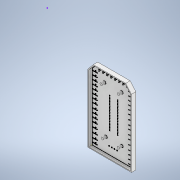
# Autodesk Inventor part: CaseV1
Saved by Autodesk Inventor 2021 (Build 250183000, 183)
## iProperties
Created: 2021-02-27
Part Number: CaseV1
Material: ABS Plastic
Document SubType Name: Modeling
Designer: Collin
Density: 1.06 g/cm^3
Appearance: Smooth - White
Mass: 45.9526 g
Surface Area: 316.416 cm^2
Volume: 43.3515 cm^3
Author: Collin
Autodesk Inventor part; units mm, degrees
ref_plane "YZ Plane" through (0, 0, 0) normal (1, 0, 0) x (0, 1, 0)
ref_plane "XZ Plane" through (0, 0, 0) normal (0, 1, 0) x (-1, 0, 0)
ref_plane "XY Plane" through (0, 0, 0) normal (0, 0, 1) x (1, 0, 0)
sketch "Sketch1" plane through (0, 0, 0) normal (0, 0, 1) x (1, 0, 0)
  line L0 (79.756, 127.254) -> (79.756, 0)
  line L1 (69.85, 138.938) -> (79.756, 127.254)
  line L2 (9.398, 138.938) -> (69.85, 138.938)
  line L3 (0, 127.762) -> (9.398, 138.938)
  line L4 (0, 0) -> (0, 127.762)
  line L5 (79.756, 0) -> (0, 0)
  circle A0 centre (28.448, 132.08) radius 0.51
  circle A1 centre (20.828, 132.08) radius 0.51
  circle A2 centre (22.988, 132.08) radius 0.55
  circle A3 centre (23.368, 115.57) radius 2.54
  circle A4 centre (13.208, 129.54) radius 0.51
  circle A5 centre (6.858, 101.6) radius 0.51
  circle A6 centre (9.398, 101.6) radius 0.51
  circle A7 centre (6.858, 103.76) radius 0.55
  circle A8 centre (9.398, 109.22) radius 0.51
  circle A9 centre (6.858, 109.22) radius 0.51
  circle A10 centre (6.858, 111.38) radius 0.55
  circle A11 centre (6.858, 124.46) radius 0.51
  circle A12 centre (9.398, 124.46) radius 0.51
  circle A13 centre (9.398, 116.84) radius 0.51
  circle A14 centre (6.858, 116.84) radius 0.51
  circle A15 centre (6.858, 119) radius 0.55
  circle A16 centre (6.858, 126.62) radius 0.55
  circle A17 centre (6.858, 96.14) radius 0.55
  circle A18 centre (6.858, 88.52) radius 0.55
  circle A19 centre (9.398, 93.98) radius 0.51
  circle A20 centre (6.858, 93.98) radius 0.51
  circle A21 centre (6.858, 39.37) radius 0.51
  circle A22 centre (6.858, 41.53) radius 0.55
  circle A23 centre (6.858, 49.15) radius 0.55
  circle A24 centre (6.858, 46.99) radius 0.51
  circle A25 centre (6.858, 54.61) radius 0.51
  circle A26 centre (6.858, 56.77) radius 0.55
  circle A27 centre (6.858, 80.9) radius 0.55
  circle A28 centre (6.858, 78.74) radius 0.51
  circle A29 centre (6.858, 73.28) radius 0.55
  circle A30 centre (6.858, 64.39) radius 0.55
  circle A31 centre (6.858, 71.12) radius 0.51
  circle A32 centre (6.858, 62.23) radius 0.51
  circle A33 centre (9.398, 71.12) radius 0.51
  circle A34 centre (9.398, 62.23) radius 0.51
  circle A35 centre (9.398, 39.37) radius 0.51
  circle A36 centre (9.398, 46.99) radius 0.51
  circle A37 centre (9.398, 54.61) radius 0.51
  circle A38 centre (9.398, 78.74) radius 0.51
  circle A39 centre (6.858, 86.36) radius 0.51
  circle A40 centre (9.398, 86.36) radius 0.51
  circle A41 centre (1.778, 78.74) radius 0.51
  circle A42 centre (1.778, 86.36) radius 0.51
  circle A43 centre (1.778, 109.22) radius 0.51
  circle A44 centre (1.778, 101.6) radius 0.51
  circle A45 centre (1.778, 93.98) radius 0.51
  circle A46 centre (4.318, 78.74) radius 0.51
  circle A47 centre (4.318, 86.36) radius 0.51
  circle A48 centre (4.318, 109.22) radius 0.51
  circle A49 centre (4.318, 101.6) radius 0.51
  circle A50 centre (4.318, 93.98) radius 0.51
  circle A51 centre (4.318, 39.37) radius 0.51
  circle A52 centre (1.778, 39.37) radius 0.51
  circle A53 centre (1.778, 54.61) radius 0.51
  circle A54 centre (4.318, 54.61) radius 0.51
  circle A55 centre (4.318, 46.99) radius 0.51
  circle A56 centre (1.778, 46.99) radius 0.51
  circle A57 centre (1.778, 71.12) radius 0.51
  circle A58 centre (4.318, 71.12) radius 0.51
  circle A59 centre (1.778, 62.23) radius 0.51
  circle A60 centre (4.318, 62.23) radius 0.51
  circle A61 centre (4.318, 124.46) radius 0.51
  circle A62 centre (4.318, 116.84) radius 0.51
  circle A63 centre (1.778, 116.84) radius 0.51
  circle A64 centre (1.778, 124.46) radius 0.51
  circle A65 centre (33.528, 40.64) radius 0.5
  circle A66 centre (36.068, 137.16) radius 0.51
  circle A67 centre (36.068, 134.62) radius 0.51
  circle A68 centre (36.068, 132.08) radius 0.51
  circle A69 centre (36.068, 129.54) radius 0.51
  circle A70 centre (33.528, 76.2) radius 0.5
  circle A71 centre (33.528, 78.74) radius 0.5
  circle A72 centre (33.528, 81.28) radius 0.5
  circle A73 centre (33.528, 88.9) radius 0.5
  circle A74 centre (33.528, 86.36) radius 0.5
  circle A75 centre (33.528, 83.82) radius 0.5
  circle A76 centre (33.528, 93.98) radius 0.5
  circle A77 centre (33.528, 91.44) radius 0.5
  circle A78 centre (33.528, 96.52) radius 0.5
  circle A79 centre (33.528, 99.06) radius 0.5
  circle A80 centre (33.528, 45.72) radius 0.5
  circle A81 centre (33.528, 48.26) radius 0.5
  circle A82 centre (33.528, 53.34) radius 0.5
  circle A83 centre (33.528, 50.8) radius 0.5
  circle A84 centre (33.528, 58.42) radius 0.5
  circle A85 centre (33.528, 55.88) radius 0.5
  circle A86 centre (33.528, 73.66) radius 0.5
  circle A87 centre (33.528, 71.12) radius 0.5
  circle A88 centre (33.528, 68.58) radius 0.5
  circle A89 centre (33.528, 63.5) radius 0.5
  circle A90 centre (33.528, 66.04) radius 0.5
  circle A91 centre (33.528, 60.96) radius 0.5
  circle A92 centre (30.608, 132.08) radius 0.55
  circle A93 centre (33.528, 43.18) radius 0.5
  circle A94 centre (13.208, 134.62) radius 0.51
  circle A95 centre (20.828, 134.62) radius 0.51
  circle A96 centre (15.368, 132.08) radius 0.55
  circle A97 centre (13.208, 132.08) radius 0.51
  circle A98 centre (20.828, 129.54) radius 0.51
  circle A99 centre (13.208, 137.16) radius 0.51
  circle A100 centre (20.828, 137.16) radius 0.51
  circle A101 centre (28.448, 137.16) radius 0.51
  circle A102 centre (28.448, 134.62) radius 0.51
  circle A103 centre (28.448, 129.54) radius 0.51
  circle A104 centre (77.978, 44.45) radius 0.51
  circle A105 centre (75.438, 46.61) radius 0.55
  circle A106 centre (75.438, 44.45) radius 0.51
  circle A107 centre (75.438, 54.23) radius 0.55
  circle A108 centre (75.438, 52.07) radius 0.51
  circle A109 centre (77.978, 52.07) radius 0.51
  circle A110 centre (77.978, 60.96) radius 0.51
  circle A111 centre (75.438, 60.96) radius 0.51
  circle A112 centre (75.438, 63.12) radius 0.55
  circle A113 centre (70.358, 52.07) radius 0.51
  circle A114 centre (70.358, 44.45) radius 0.51
  circle A115 centre (70.358, 60.96) radius 0.51
  circle A116 centre (72.898, 60.96) radius 0.51
  circle A117 centre (72.898, 44.45) radius 0.51
  circle A118 centre (72.898, 52.07) radius 0.51
  circle A119 centre (70.358, 68.326) radius 0.51
  circle A120 centre (72.898, 68.326) radius 0.51
  circle A121 centre (77.978, 68.326) radius 0.51
  circle A122 centre (75.438, 68.326) radius 0.51
  circle A123 centre (75.438, 79.376) radius 0.55
  circle A124 centre (75.438, 77.216) radius 0.51
  circle A125 centre (77.978, 77.216) radius 0.51
  circle A126 centre (75.438, 70.486) radius 0.55
  circle A127 centre (72.898, 77.216) radius 0.51
  circle A128 centre (70.358, 77.216) radius 0.51
  circle A129 centre (48.768, 78.74) radius 0.5
  circle A130 centre (48.768, 76.2) radius 0.5
  circle A131 centre (48.768, 73.66) radius 0.5
  circle A132 centre (48.768, 68.58) radius 0.5
  circle A133 centre (48.768, 71.12) radius 0.5
  circle A134 centre (48.768, 66.04) radius 0.5
  circle A135 centre (48.768, 50.8) radius 0.5
  circle A136 centre (48.768, 53.34) radius 0.5
  circle A137 centre (48.768, 58.42) radius 0.5
  circle A138 centre (48.768, 55.88) radius 0.5
  circle A139 centre (48.768, 63.5) radius 0.5
  circle A140 centre (48.768, 60.96) radius 0.5
  circle A141 centre (48.768, 48.26) radius 0.5
  circle A142 centre (48.768, 45.72) radius 0.5
  circle A143 centre (75.438, 103.506) radius 0.55
  circle A144 centre (75.438, 101.346) radius 0.51
  circle A145 centre (72.898, 101.346) radius 0.51
  circle A146 centre (75.438, 95.886) radius 0.55
  circle A147 centre (72.898, 86.106) radius 0.51
  circle A148 centre (75.438, 88.266) radius 0.55
  circle A149 centre (75.438, 86.106) radius 0.51
  circle A150 centre (75.438, 93.726) radius 0.51
  circle A151 centre (72.898, 93.726) radius 0.51
  circle A152 centre (70.358, 93.726) radius 0.51
  circle A153 centre (70.358, 101.346) radius 0.51
  circle A154 centre (70.358, 86.106) radius 0.51
  circle A155 centre (48.768, 86.36) radius 0.5
  circle A156 centre (48.768, 88.9) radius 0.5
  circle A157 centre (48.768, 91.44) radius 0.5
  circle A158 centre (48.768, 96.52) radius 0.5
  circle A159 centre (48.768, 93.98) radius 0.5
  circle A160 centre (48.768, 99.06) radius 0.5
  circle A161 centre (77.978, 93.726) radius 0.51
  circle A162 centre (77.978, 86.106) radius 0.51
  circle A163 centre (77.978, 101.346) radius 0.51
  circle A164 centre (48.768, 83.82) radius 0.5
  circle A165 centre (48.768, 81.28) radius 0.5
  circle A166 centre (66.548, 129.54) radius 0.51
  circle A167 centre (58.928, 129.54) radius 0.51
  circle A168 centre (51.308, 129.54) radius 0.51
  circle A169 centre (70.358, 123.952) radius 0.51
  circle A170 centre (72.898, 116.586) radius 0.51
  circle A171 centre (70.358, 116.586) radius 0.51
  circle A172 centre (72.898, 123.952) radius 0.51
  circle A173 centre (56.388, 115.57) radius 2.54
  circle A174 centre (77.978, 116.586) radius 0.51
  circle A175 centre (75.438, 116.586) radius 0.51
  circle A176 centre (75.438, 118.746) radius 0.55
  circle A177 centre (75.438, 126.112) radius 0.55
  circle A178 centre (75.438, 123.952) radius 0.51
  circle A179 centre (77.978, 123.952) radius 0.51
  circle A180 centre (75.438, 108.966) radius 0.51
  circle A181 centre (77.978, 108.966) radius 0.51
  circle A182 centre (72.898, 108.966) radius 0.51
  circle A183 centre (75.438, 111.126) radius 0.55
  circle A184 centre (70.358, 108.966) radius 0.51
  circle A185 centre (51.308, 137.16) radius 0.51
  circle A186 centre (51.308, 134.62) radius 0.51
  circle A187 centre (58.928, 137.16) radius 0.51
  circle A188 centre (58.928, 134.62) radius 0.51
  circle A189 centre (66.548, 134.62) radius 0.51
  circle A190 centre (66.548, 137.16) radius 0.51
  circle A191 centre (53.468, 132.08) radius 0.55
  circle A192 centre (61.088, 132.08) radius 0.55
  circle A193 centre (58.928, 132.08) radius 0.51
  circle A194 centre (51.308, 132.08) radius 0.51
  circle A195 centre (66.548, 132.08) radius 0.51
  circle A196 centre (68.708, 132.08) radius 0.55
  circle A197 centre (43.688, 129.54) radius 0.51
  circle A198 centre (43.688, 132.08) radius 0.51
  circle A199 centre (43.688, 134.62) radius 0.51
  circle A200 centre (45.848, 132.08) radius 0.55
  circle A201 centre (43.688, 137.16) radius 0.51
  circle A202 centre (48.768, 43.18) radius 0.5
  circle A203 centre (38.228, 132.08) radius 0.55
  circle A204 centre (48.768, 40.64) radius 0.5
  circle A205 centre (4.318, 12.7) radius 0.51
  circle A206 centre (6.858, 14.86) radius 0.55
  circle A207 centre (6.858, 12.7) radius 0.51
  circle A208 centre (9.398, 12.7) radius 0.51
  circle A209 centre (32.258, 14.732) radius 0.89
  circle A210 centre (37.338, 14.732) radius 0.89
  circle A211 centre (77.978, 19.05) radius 0.51
  circle A212 centre (75.438, 19.05) radius 0.51
  circle A213 centre (75.438, 13.59) radius 0.55
  circle A214 centre (70.358, 19.05) radius 0.51
  circle A215 centre (72.898, 19.05) radius 0.51
  circle A216 centre (42.418, 14.732) radius 0.89
  circle A217 centre (47.498, 14.732) radius 0.89
  circle A218 centre (4.318, 21.59) radius 0.51
  circle A219 centre (6.858, 21.59) radius 0.51
  circle A220 centre (9.398, 21.59) radius 0.51
  circle A221 centre (9.398, 30.48) radius 0.51
  circle A222 centre (25.908, 26.67) radius 2.54
  circle A223 centre (77.978, 26.67) radius 0.51
  circle A224 centre (75.438, 26.67) radius 0.51
  circle A225 centre (70.358, 26.67) radius 0.51
  circle A226 centre (72.898, 26.67) radius 0.51
  circle A227 centre (75.438, 28.83) radius 0.55
  circle A228 centre (56.388, 26.67) radius 2.5527
  circle A229 centre (75.438, 21.21) radius 0.55
  circle A230 centre (4.318, 30.48) radius 0.51
  circle A231 centre (6.858, 30.48) radius 0.51
  circle A232 centre (6.858, 23.75) radius 0.55
  circle A233 centre (70.358, 35.56) radius 0.51
  circle A234 centre (72.898, 35.56) radius 0.51
  circle A235 centre (77.978, 35.56) radius 0.51
  circle A236 centre (75.438, 35.56) radius 0.51
  circle A237 centre (6.858, 32.64) radius 0.55
  circle A238 centre (1.778, 30.48) radius 0.51
  circle A239 centre (1.778, 21.59) radius 0.51
  circle A240 centre (1.778, 12.7) radius 0.51
  circle A241 centre (75.438, 37.72) radius 0.55
  circle A242 centre (72.898, 3.81) radius 0.51
  circle A243 centre (77.978, 3.81) radius 0.51
  circle A244 centre (75.438, 3.81) radius 0.51
  circle A245 centre (75.438, 5.97) radius 0.55
  circle A246 centre (70.358, 3.81) radius 0.51
  circle A247 centre (6.858, 7.24) radius 0.55
  circle A248 centre (6.858, 5.08) radius 0.51
  circle A249 centre (9.398, 5.08) radius 0.51
  circle A250 centre (1.778, 5.08) radius 0.51
  circle A251 centre (4.318, 5.08) radius 0.51
  circle A252 centre (75.438, 11.43) radius 0.51
  circle A253 centre (72.898, 11.43) radius 0.51
  circle A254 centre (70.358, 11.43) radius 0.51
  circle A255 centre (77.978, 11.43) radius 0.51
  point P0 (-85.852, 184.15)
  constraints: 256 centre point, 250 equal radius, 12 end point, 3 horizontal, 3 vertical, 2 parallel, 521 other
sketch "Sketch2" plane through (0, 0, 0) normal (0, 0, 1) x (1, 0, 0)
  circle A0 centre (23.368, 115.57) radius 2.54 projected
  circle A1 centre (56.388, 115.57) radius 2.54 projected
  line L0 (0, 127.762) -> (9.398, 138.938) projected
  line L1 (9.398, 138.938) -> (69.85, 138.938) projected
  line L2 (0, 0) -> (0, 127.762) projected
  line L3 (69.85, 138.938) -> (79.756, 127.254) projected
  line L4 (79.756, 127.254) -> (79.756, 0) projected
  line L5 (79.756, 0) -> (0, 0) projected
  circle A2 centre (25.908, 26.67) radius 2.54 projected
  circle A3 centre (56.388, 26.67) radius 2.5527 projected
  circle A4 centre (23.368, 115.57) radius 2.286
  circle A5 centre (56.388, 115.57) radius 2.286
  circle A6 centre (25.908, 26.67) radius 2.286
  circle A7 centre (56.388, 26.67) radius 2.286
  line L6 (-0.254, 127.8546) -> (9.2797, 139.192)
  line L7 (9.2797, 139.192) -> (69.9677, 139.192)
  line L8 (69.9677, 139.192) -> (80.01, 127.3472)
  line L9 (80.01, 127.3472) -> (80.01, -0.254)
  line L10 (80.01, -0.254) -> (-0.254, -0.254)
  line L11 (-0.254, -0.254) -> (-0.254, 127.8546)
  line L12 (8.5405, 140.7795) -> (-1.8415, 128.4334)
  line L13 (-1.8415, 128.4334) -> (-1.8415, -1.8415)
  line L14 (-1.8415, -1.8415) -> (81.5975, -1.8415)
  line L15 (81.5975, -1.8415) -> (81.5975, 127.9296)
  line L16 (81.5975, 127.9296) -> (70.703, 140.7795)
  line L17 (70.703, 140.7795) -> (8.5405, 140.7795)
  dimension "d528" = 0.254
  dimension "d532" = 0.254
  dimension "d533" = 1.5875
  constraints: 24 end point, 4 centre point, 3 equal radius, 10 other
  measures "d528" radial gap between concentric circles of A0 A4
  measures "d532" distance between parallel lines of L2 L11
  measures "d533" distance between parallel lines of L6 L12
extrude "Extrusion1" add sketch "Sketch2" along normal blind 6.35 contours A4 | A5 | A6 | A7 | L17 L16 L15 L14 L13 L12
sketch "Sketch4" plane through (0, 0, 0) normal (0, 0, -1) x (-1, 0, 0)
  line L0 (1.8415, 128.4334) -> (1.8415, -1.8415) projected
  line L1 (-8.5405, 140.7795) -> (1.8415, 128.4334) projected
  line L2 (-70.703, 140.7795) -> (-8.5405, 140.7795) projected
  line L3 (-81.5975, 127.9296) -> (-70.703, 140.7795) projected
  line L4 (-81.5975, -1.8415) -> (-81.5975, 127.9296) projected
  line L5 (1.8415, -1.8415) -> (-81.5975, -1.8415) projected
  line L6 (0.254, 127.8546) -> (-9.2797, 139.192) projected
  line L7 (0.254, -0.254) -> (0.254, 127.8546) projected
  line L8 (-80.01, -0.254) -> (0.254, -0.254) projected
  line L9 (-80.01, 127.3472) -> (-80.01, -0.254) projected
  line L10 (-69.9677, 139.192) -> (-80.01, 127.3472) projected
  line L11 (-9.2797, 139.192) -> (-69.9677, 139.192) projected
  point P0 (0, 0)
extrude "Extrusion3" add sketch "Sketch4" along normal blind 2.032 contours L0 L5 L4 L3 L2 L1 | L7 L8 L9 L10 L11 L6
body "Solid1"
